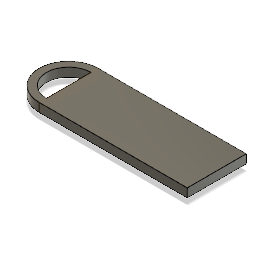
cyka blyat v0 (Autodesk Fusion 360 design; units mm, degrees)
Autodesk Fusion 360 part; units mm, degrees
sketch "草图1" plane through (0, 0, 0) normal (0, 1, 0) x (1, 0, 0)
  line L0 (0, 0) -> (50, 0)
  line L1 (50, 0) -> (50, -20)
  line L2 (50, -20) -> (0, -20)
  line L3 (0, -20) -> (0, 0)
  dimension "d1" = 50
  dimension "d2" = 20
extrude "拉伸1" add sketch "草图1" along normal blind 3
sketch "草图2" plane through (0, 0, 0) normal (-1, 0, 0) x (0, 0, 1)
  line L0 (0, 0) -> (20, 0)
  line L1 (20, 0) -> (20, 3)
  line L2 (20, 3) -> (0, 3)
  line L3 (0, 3) -> (0, 0)
sketch "草图3" plane through (0, 3, 0) normal (0, 1, 0) x (-1, 0, 0)
  line L0 (0, 20) -> (-50, 20)
  line L1 (-50, 20) -> (-50, 0)
  line L2 (-50, 0) -> (0, 0)
  line L3 (0, 0) -> (0, 20)
  arc A0 (0, 0) -> (0, 20) centre (0, 10) ccw
  arc A1 (0, 2.5) -> (0, 17.5) centre (0, 10) ccw
  dimension "d5" = 2.5
extrude "拉伸2" add sketch "草图3" against normal blind 3 contours L3 A0 A1
sketch "草图4" plane through (0, 0, 0) normal (0, 1, 0) x (1, 0, 0)
  line L0 (3, -5) -> (46.999, -5) construction
  line L1 (46.999, -5) -> (46.999, -15) construction
  line L2 (46.999, -15) -> (3, -15) construction
  line L3 (3, -15) -> (3, -5) construction
  text T0 "cyka blyat" font "Arial" height 10 align ink ink in box 0 x 0 at (3, -5) x (1, 0) y (0, -1) spacing 1 kerned height is em
extrude "拉伸3" add sketch "草图4" against normal blind 2 text T0
